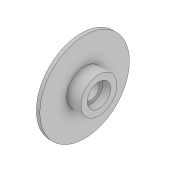
# Autodesk Inventor part: Reel1ACABARMEDIDAS
Saved by Autodesk Inventor 2022 (Build 260153000, 153)
## iProperties
Created: 2019-08-23
Part Number: Reel1ACABARMEDIDAS
Material: Genérico
Document SubType Name: Modeling
Designer: Cristiano
Density: 1 g/cm^3
Appearance: Valor por defecto
Author: Cristiano
Autodesk Inventor part; units mm, degrees
ref_plane "YZ Plane" through (0, 0, 0) normal (1, 0, 0) x (0, 1, 0)
ref_plane "XZ Plane" through (0, 0, 0) normal (0, 1, 0) x (-1, 0, 0)
ref_plane "XY Plane" through (0, 0, 0) normal (0, 0, 1) x (1, 0, 0)
sketch "Boceto1" plane through (0, 0, 0) normal (0, 0, 1) x (1, 0, 0)
  line L0 (0, 0) -> (24.2042, 0) construction
  line L1 (0, 9.5) -> (11, 9.5)
  line L2 (0, 9.5) -> (0, 50)
  line L3 (0, 50) -> (4, 50)
  line L4 (4, 50) -> (4, 20)
  line L5 (4, 20) -> (20, 20)
  line L6 (20, 20) -> (20, 13.925)
  line L7 (20, 13.925) -> (11, 13.925)
  line L8 (11, 13.925) -> (11, 9.5)
  line L9 (0, 0) -> (0, 63.5344) construction
  line L10 (10.3397, 15) -> (10.3397, 20) construction
  line L11 (10.3397, 20) -> (20, 20) construction
  dimension "d0" = 50
  dimension "d1" = 4
  dimension "d4" = 13.925
  dimension "d10" = 9.5
  dimension "d11" = 9
  dimension "d13" = 20
  dimension "d15" = 20
  constraints: 25 end point, 6 perpendicular, 3 vertical, 2 horizontal, 1 collinear
  measures "d0" distance between parallel lines of L0 L3
  measures "d1" distance of L2.end L3.end
  measures "d4" distance between parallel lines of L0 L7
  measures "d10" distance between parallel lines of L0 L1
  measures "d11" distance of L6.end L7.end
  measures "d13" distance from line of L0 L10.end
  measures "d15" distance between parallel lines of L6 L2
revolve "Revolución1" add sketch "Boceto1" angle 360 about axis through (0, 0, 0) along (1, 0, 0)
sketch "Sketch2" plane through (20, 0, 0) normal (1, 0, 0) x (0, 0, -1)
  circle A0 centre (0, 0) radius 13
  circle A1 centre (0, 0) radius 13.925 projected
  dimension "d16" = 26
  constraints: 1 centre point, 1 coincident
  measures "d16" diameter of A0
extrude "Extrusion1" add sketch "Sketch2" against normal up to surface (9 mm away)
